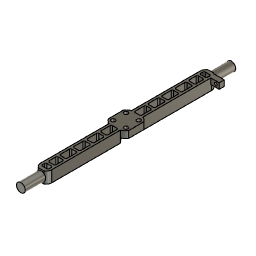
Motor_Mounts (Autodesk Fusion 360 design; units mm, degrees)
Autodesk Fusion 360 part; units mm, degrees
note: some values were not read from the file. Set by a fixed rule: which sketch regions a step uses.
sketch "Sketch1" plane through (0, 0, 0) normal (0, 0, 1) x (1, 0, 0)
  line L0 (-9, -10) -> (9, -10)
  line L1 (9, -10) -> (9, 10)
  line L2 (9, 10) -> (-9, 10)
  line L3 (-9, 10) -> (-9, -10)
  circle A0 centre (0, -8) radius 1.75
  circle A1 centre (5.6569, -5.6569) radius 1.75
  circle A2 centre (8, 0) radius 1.75
  circle A3 centre (5.6569, 5.6569) radius 1.75
  circle A4 centre (0, 8) radius 1.75
  circle A5 centre (-5.6569, 5.6569) radius 1.75
  circle A6 centre (-8, 0) radius 1.75
  circle A7 centre (-5.6569, -5.6569) radius 1.75
  line L4 (-5, -10) -> (-3, -10)
  line L5 (-3, -10) -> (-3, -66)
  line L6 (-3, -66) -> (-5, -66)
  line L7 (-5, -66) -> (-5, -10)
  line L8 (3, -10) -> (5, -10)
  line L9 (5, -10) -> (5, -66)
  line L10 (5, -66) -> (3, -66)
  line L11 (3, -66) -> (3, -10)
  line L12 (-3, -20) -> (3, -20)
  line L13 (3, -20) -> (3, -22)
  line L14 (3, -22) -> (-3, -22)
  line L15 (-3, -22) -> (-3, -20)
  line L16 (-3, -32) -> (3, -32)
  line L17 (3, -32) -> (3, -34)
  line L18 (3, -34) -> (-3, -34)
  line L19 (-3, -34) -> (-3, -32)
  line L20 (-3, -44) -> (3, -44)
  line L21 (3, -44) -> (3, -46)
  line L22 (3, -46) -> (-3, -46)
  line L23 (-3, -46) -> (-3, -44)
  line L24 (-3, -56) -> (3, -56)
  line L25 (3, -56) -> (3, -58)
  line L26 (3, -58) -> (-3, -58)
  line L27 (-3, -58) -> (-3, -56)
  line L28 (20, 0) -> (2.5, 0)
  line L29 (-3, 56) -> (3, 56)
  line L30 (3, 46) -> (-3, 46)
  line L31 (-3, 22) -> (-3, 20)
  line L32 (-5, 10) -> (-3, 10)
  line L33 (3, 58) -> (-3, 58)
  line L34 (-3, 34) -> (-3, 32)
  line L35 (3, 34) -> (-3, 34)
  line L36 (3, 66) -> (3, 10)
  line L37 (-3, 44) -> (3, 44)
  line L38 (-3, 46) -> (-3, 44)
  line L39 (3, 10) -> (5, 10)
  line L40 (-3, 66) -> (-5, 66)
  line L41 (5, 10) -> (5, 66)
  line L42 (-3, 32) -> (3, 32)
  line L43 (-5, 66) -> (-5, 10)
  line L44 (3, 56) -> (3, 58)
  line L45 (5, 66) -> (3, 66)
  line L46 (3, 22) -> (-3, 22)
  line L47 (3, 32) -> (3, 34)
  line L48 (-3, 58) -> (-3, 56)
  line L49 (3, 44) -> (3, 46)
  line L50 (-3, 10) -> (-3, 66)
  line L51 (-3, 20) -> (3, 20)
  line L52 (3, 20) -> (3, 22)
  circle A8 centre (0, 0) radius 11.25
  dimension "d1" = 9
  dimension "d2" = 18
  dimension "d3" = 20
  dimension "d4" = 10
  dimension "d5" = 3.5
  dimension "d6" = 8
  dimension "d7" = 9
  dimension "d9" = 360
  dimension "d10" = 2
  dimension "d11" = 2
  dimension "d12" = 6
  dimension "d13" = 3
  dimension "d14" = 56
  dimension "d15" = 56
  dimension "d16" = 10
  dimension "d17" = 2
  dimension "d18" = 10
  dimension "d19" = 2
  dimension "d20" = 10
  dimension "d21" = 2
  dimension "d22" = 10
  dimension "d23" = 2
  dimension "d29" = 22.5
  constraint horizontal L0
  constraint vertical L1
  constraint horizontal L2
  constraint vertical L3
  constraint horizontal L4
  constraint vertical L5
  constraint horizontal L6
  constraint vertical L7
  constraint coincident L0 L4.start
  constraint horizontal L8
  constraint vertical L9
  constraint horizontal L10
  constraint vertical L11
  constraint coincident L0 L8.start
  constraint horizontal L12
  constraint vertical L13
  constraint horizontal L14
  constraint vertical L15
  constraint coincident L11 L13.end
  constraint coincident L5 L12.start
  constraint horizontal L16
  constraint vertical L17
  constraint horizontal L18
  constraint vertical L19
  constraint coincident L11 L17.end
  constraint coincident L5 L16.start
  constraint horizontal L20
  constraint vertical L21
  constraint horizontal L22
  constraint vertical L23
  constraint coincident L11 L21.end
  constraint coincident L5 L20.start
  constraint horizontal L24
  constraint vertical L25
  constraint horizontal L26
  constraint vertical L27
  constraint coincident L11 L25.end
  constraint coincident L5 L24.start
  constraint symmetric L4.start L28 L32.start
  constraint symmetric L4.end L28 L32.end
  constraint symmetric L5.end L28 L40.start
  constraint symmetric L6.end L28 L40.end
  constraint symmetric L8.start L28 L36.end
  constraint symmetric L8.end L28 L39.end
  constraint symmetric L9.end L28 L41.end
  constraint symmetric L10.end L28 L36.start
  constraint symmetric L12.start L28 L31.end
  constraint symmetric L12.end L28 L51.end
  constraint symmetric L13.end L28 L46.start
  constraint symmetric L14.end L28 L31.start
  constraint symmetric L16.start L28 L34.end
  constraint symmetric L16.end L28 L42.end
  constraint symmetric L17.end L28 L35.start
  constraint symmetric L18.end L28 L34.start
  constraint symmetric L20.start L28 L37.start
  constraint symmetric L20.end L28 L37.end
  constraint symmetric L21.end L28 L30.start
  constraint symmetric L22.end L28 L30.end
  constraint symmetric L24.start L28 L29.start
  constraint symmetric L24.end L28 L29.end
  constraint symmetric L25.end L28 L33.start
  constraint symmetric L26.end L28 L33.end
  constraint coincident A8.centre origin
  measures "d1" distance of A8.centre L1
  measures "d2" distance of L1 L3
  measures "d3" distance of L0 L2
  measures "d4" distance of A8.centre L0
  measures "d5" diameter of A0
  measures "d6" vertical distance of A8.centre A0.centre
  measures "d7" distance of L1 A0.centre
  measures "d10" distance of L5 L7
  measures "d11" distance of L9 L11
  measures "d12" distance of L5 L11
  measures "d13" distance of A0.centre L5
  measures "d14" distance of L4 L6
  measures "d15" distance of L0 L10
  measures "d16" distance of L0 L12
  measures "d17" distance of L12 L14
  measures "d18" distance of L14 L16
  measures "d19" distance of L16 L18
  measures "d20" distance of L18 L20
  measures "d21" distance of L20 L22
  measures "d22" distance of L22 L24
  measures "d23" distance of L24 L26
  measures "d29" diameter of A8
extrude "Extrude1" add sketch "Sketch1" along normal blind 10 contours L0 L4 L5 L7 A8 | L5 L6 L7 L15 L19 L23 L27 A8 | L0 L8 L9 L11 A8 | L9 L10 L11 L13 L17 L21 L25 A8 | L5 L11 L12 L13 L14 L15 | L5 L11 L24 L25 L26 L27 | L5 L11 L16 L17 L18 L19 | L2 L32 L43 L50 A8 | L31 L34 L38 L40 L43 L48 L50 A8 | L5 L11 L20 L21 L22 L23 | L2 L36 L39 L41 A8 | L31 L36 L46 L50 L51 L52 | L36 L41 L44 L45 L47 L49 L52 A8 | L29 L33 L36 L44 L48 L50 | L34 L35 L36 L42 L47 L50 | L30 L36 L37 L38 L49 L50 makes body 1 at (-5, -47.3333, 3.3333) makes body 2 at (5, 28.6667, 3.3333)
extrude "Extrude2" add sketch "Sketch1" along normal blind 6 from surface at 4 contours L0 L1 L2 L3 A2 A6 L4 L8 L32 L39 A8 | L3 A6 | L1 A2 L28 | L1 A2 L28 | A0 | A4 picked at (-8.2184, 0.4897) picked at (7.1728, -0.0844) picked at (7.1728, 0.0844) bodies 1 2
sketch "Sketch2" plane through (0, 0, 10) normal (0, 0, 1) x (-1, 0, 0)
  line L0 (5, 10) -> (5, 66)
  line L1 (5, 66) -> (3, 66)
  line L2 (3, 66) -> (3, 58)
  line L3 (3, 58) -> (-3, 58)
  line L4 (-3, 58) -> (-3, 66)
  line L5 (-3, 66) -> (-5, 66)
  line L6 (-5, 66) -> (-5, 10)
  line L7 (-5, 10) -> (-5.1539, 10)
  arc A0 (-5.1539, 10) -> (-9, 6.75) centre (0, 0) ccw
  line L8 (-9, 6.75) -> (-9, -6.75)
  arc A1 (-9, -6.75) -> (-5.1539, -10) centre (0, 0) ccw
  line L9 (-5.1539, -10) -> (-5, -10)
  line L10 (-5, -10) -> (-5, -66)
  line L11 (-5, -66) -> (-3, -66)
  line L12 (-3, -66) -> (-3, -58)
  line L13 (-3, -58) -> (3, -58)
  line L14 (3, -58) -> (3, -66)
  line L15 (3, -66) -> (5, -66)
  line L16 (5, -66) -> (5, -10)
  line L17 (5, -10) -> (5.1539, -10)
  arc A2 (5.1539, -10) -> (9, -6.75) centre (0, 0) ccw
  line L18 (9, -6.75) -> (9, 6.75)
  arc A3 (9, 6.75) -> (5.1539, 10) centre (0, 0) ccw
  line L19 (5.1539, 10) -> (5, 10)
  line L20 (-3, -44) -> (-3, -34)
  line L21 (-3, -34) -> (3, -34)
  line L22 (3, -34) -> (3, -44)
  line L23 (3, -44) -> (-3, -44)
  line L24 (-3, -56) -> (-3, -46)
  line L25 (-3, -46) -> (3, -46)
  line L26 (3, -46) -> (3, -56)
  line L27 (3, -56) -> (-3, -56)
  line L28 (-3, -32) -> (-3, -22)
  line L29 (-3, -22) -> (3, -22)
  line L30 (3, -22) -> (3, -32)
  line L31 (3, -32) -> (-3, -32)
  circle A4 centre (5.6569, 5.6569) radius 1.75
  circle A5 centre (5.6569, -5.6569) radius 1.75
  circle A6 centre (-5.6569, -5.6569) radius 1.75
  circle A7 centre (-5.6569, 5.6569) radius 1.75
  line L32 (3, -10) -> (3, -20)
  line L33 (3, -20) -> (-3, -20)
  line L34 (-3, -20) -> (-3, -10)
  line L35 (-3, -10) -> (3, -10)
  line L36 (-3, 32) -> (3, 32)
  line L37 (3, 32) -> (3, 22)
  line L38 (3, 22) -> (-3, 22)
  line L39 (-3, 22) -> (-3, 32)
  line L40 (-3, 56) -> (3, 56)
  line L41 (3, 56) -> (3, 46)
  line L42 (3, 46) -> (-3, 46)
  line L43 (-3, 46) -> (-3, 56)
  line L44 (-3, 44) -> (3, 44)
  line L45 (3, 44) -> (3, 34)
  line L46 (3, 34) -> (-3, 34)
  line L47 (-3, 34) -> (-3, 44)
  line L48 (3, 10) -> (-3, 10)
  line L49 (-3, 10) -> (-3, 20)
  line L50 (-3, 20) -> (3, 20)
  line L51 (3, 20) -> (3, 10)
  line L52 (5, 10) -> (0.642, 5.0534)
  line L53 (0.642, 5.0534) -> (0.642, -4.9902)
  line L54 (0.642, -4.9902) -> (5, -10)
  line L55 (3, -10) -> (0, -6.5513)
  line L56 (0, -6.5513) -> (-3, -10)
  line L57 (-5.1539, -10) -> (-0.8022, -4.9974)
  line L58 (-0.8022, -4.9974) -> (-0.8022, 5.117)
  line L59 (-0.8022, 5.117) -> (-5, 10)
  line L60 (-3, 10) -> (0, 6.5103)
  line L61 (0, 6.5103) -> (3, 10)
  line L62 (5, 10) -> (3, 10)
  line L63 (-3, 10) -> (-5, 10)
  line L64 (-3, -10) -> (-5.1539, -10)
  line L65 (3, -10) -> (5, -10)
  constraint coincident L0.start L19.end
  constraint perpendicular L7 L53
  constraint coincident L16.end L17.start
  constraint coincident L32.start L35.end
  constraint parallel L54 L55
  constraint coincident L34.end L35.start
  constraint coincident A1.end L9.start
  constraint parallel L56 L57
  constraint parallel L10 L58
  constraint coincident L6.end L7.start
  constraint coincident L48.end L49.start
  constraint parallel L59 L60
  constraint coincident L48.start L51.end
extrude "Extrude3" add sketch "Sketch2" against normal blind 4 from surface at -6 contours L9 L52 L53 L54 L55 L56 L57 L58 L59 L60 L61 L62 L63 L64 L65 bodies 1
sketch "Sketch3" plane through (0, 0, 0) normal (0, 0, 1) x (1, 0, 0)
  line L0 (-5, 66) -> (5, 66)
  line L1 (5, 66) -> (5, 70.6982)
  line L2 (2.5484, 75) -> (-2.5484, 75)
  line L3 (-5, 70.6982) -> (-5, 66)
  line L4 (-3, 68) -> (3, 68)
  line L5 (3, 68) -> (3, 72)
  line L6 (3, 72) -> (-3, 72)
  line L7 (-3, 72) -> (-3, 68)
  arc A0 (5, 70.6982) -> (2.5484, 75) centre (0, 70.6982) ccw
  arc A1 (-2.5484, 75) -> (-5, 70.6982) centre (0, 70.6982) ccw
  line L8 (20, 0) -> (2.5, 0)
  arc A2 (-5, -70.6982) -> (-2.5484, -75) centre (0, -70.6982) ccw
  line L9 (3, -68) -> (3, -72)
  line L10 (2.5484, -75) -> (-2.5484, -75)
  line L11 (-3, -68) -> (3, -68)
  line L12 (5, -66) -> (5, -70.6982)
  arc A3 (2.5484, -75) -> (5, -70.6982) centre (0, -70.6982) ccw
  line L13 (-5, -70.6982) -> (-5, -66)
  line L14 (-3, -72) -> (-3, -68)
  line L15 (3, -72) -> (-3, -72)
  line L16 (-5, -66) -> (5, -66)
  point P0 (-5, 66)
  point P1 (5, 66)
  point P2 (5, -66)
  point P3 (-5, -66)
  dimension "d33" = 9
  dimension "d34" = 4.6982
  dimension "d39" = 6
  dimension "d40" = 2
  dimension "d41" = 3
  dimension "d42" = 2
  constraint horizontal L0
  constraint vertical L1
  constraint horizontal L2
  constraint vertical L3
  constraint coincident P0 L0.start
  constraint coincident P1 L0.end
  constraint horizontal L4
  constraint vertical L5
  constraint horizontal L6
  constraint vertical L7
  constraint coincident L2.end A0
  constraint concentric A0 A1
  constraint symmetric P0 L8 P3
  constraint symmetric P1 L8 L12.start
  constraint symmetric P0 L8 L13.end
  constraint symmetric P1 L8 P2
  constraint symmetric L3.start L8 A2.start
  constraint symmetric L1.end L8 L12.end
  constraint symmetric L4.start L8 L11.start
  constraint symmetric L4.end L8 L9.start
  constraint symmetric L5.end L8 L9.end
  constraint symmetric L6.end L8 L14.start
  constraint symmetric L2.end L8 A2.end
  constraint symmetric L2.start L8 L10.start
  constraint symmetric A0 L8 A3
  constraint symmetric A1 L8 A2
  measures "d33" distance of L0 L2
  measures "d34" distance of L0 A0.centre
  measures "d39" distance of L5 L7
  measures "d40" distance of L0 L4
  measures "d41" distance of L2 L6
  measures "d42" distance of L1 L5
extrude "Extrude4" add sketch "Sketch3" along normal blind 10 bodies 1
fillet "Fillet1" radius 1 22 edges at (-3, 10, 7) (-3, 20, 5) (3, 10, 7) (3, 20, 5) (3, 22, 5) (3, 32, 5) (3, 34, 5) (-3, 32, 5) (-3, 34, 5) (-3, 22, 5) (-3, 46, 5) (-3, 44, 5) (3, 46, 5) (3, 44, 5) (-3, 56, 5) (3, 56, 5) (3, 58, 5) (-3, 58, 5) (3, 68, 5) (-3, 68, 5) (-3, 72, 5) (3, 72, 5) on bodies 1
fillet "Fillet1" radius 1 24 edges at (3, -10, 7) (-3, -10, 7) (3, -20, 5) (-3, -20, 5) (3, -22, 5) (3, -32, 5) (3, -34, 5) (-3, -22, 5) (-3, -32, 5) (-3, -34, 5) (-3, -44, 5) (3, -44, 5) (3, -46, 5) (-3, -58, 5) (3, -58, 5) (3, -66, 5) (-3, -66, 5) (3, -68, 5) (3, -72, 5) (-3, -72, 5) (-3, -68, 5) (-3, -56, 5) (3, -56, 5) (-3, -46, 5) on bodies 1
fillet "Fillet1" radius 1 2 edges at (3, 66, 5) (-3, 66, 5) on bodies 1
sketch "Sketch4" plane through (0, 0, 0) normal (0, 0, 1) x (1, 0, 0)
  line L0 (3.2404, 69.8889) -> (12.4842, 69.8889)
  line L1 (3.2404, 74.3889) -> (3.2404, 69.8889)
  line L2 (12.4842, 69.8889) -> (12.4842, 74.3889)
  line L3 (12.4842, 74.3889) -> (3.2404, 74.3889)
  dimension "d53" = 4.5
  measures "d53" distance of L0.start L1.start
extrude "Extrude5" add sketch "Sketch4" along normal mid plane 5 from surface at 7.5 bodies 1
hole "Hole1" at (9.5012, 74.3889, 7.4691) direction (0, -1, 0) diameter 2.5 depth 6 tip angle 118 bodies 1
sketch "Sketch5" plane through (0, 0, 0) normal (0, 1, 0) x (1, 0, 0)
  circle A0 centre (0.0434, -5) radius 3.9
  line L0 (2.5484, 0) -> (2.5484, -10)
  line L1 (2.5484, 0) -> (-2.5484, 0)
  dimension "d61" = 2.505
  dimension "d62" = 5
  dimension "d63" = 7.8
  measures "d61" distance of A0.centre L0
  measures "d62" distance of A0.centre L1
  measures "d63" diameter of A0
extrude "Extrude6" add sketch "Sketch5" along normal blind 18 from surface at 75 bodies 1
mirror "Mirror2" about plane through (0, 0, 0) normal (0, 1, 0) of "Extrude6"
